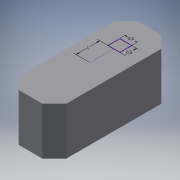
# Autodesk Inventor part: Stiftlist
Saved by Autodesk Inventor 2019 (Build 230136000, 136)
## iProperties
Created: 2018-12-16
Part Number: Stiftlist
Material: Generic
Document SubType Name: Modeling
Designer: Filip
Density: 1 g/cm^3
Appearance: Default
Author: Filip
Autodesk Inventor part; units mm, degrees
ref_plane "YZ Plane" through (0, 0, 0) normal (1, 0, 0) x (0, 1, 0)
ref_plane "XZ Plane" through (0, 0, 0) normal (0, 1, 0) x (-1, 0, 0)
ref_plane "XY Plane" through (0, 0, 0) normal (0, 0, 1) x (1, 0, 0)
sketch "Sketch1" plane through (0, 0, 0) normal (0, 1, 0) x (-1, 0, 0)
  line L0 (-1, -2.5) -> (1, -2.5)
  line L1 (1, -2.5) -> (1, 2.5)
  line L2 (1, 2.5) -> (-1, 2.5)
  line L3 (-1, 2.5) -> (-1, -2.5)
  line L4 (-1, -2.5) -> (1, 2.5) construction
  line L5 (1, -2.5) -> (-1, 2.5) construction
  point P0 (0, 0)
  dimension "d0" = 5
  dimension "d1" = 2
  constraints: 12 end point, 2 midpoint, 2 parallel, 1 horizontal, 1 perpendicular
  measures "d0" distance of L0.end L1.end
  measures "d1" distance of L1.end L2.end
extrude "Extrusion1" add sketch "Sketch1" along normal blind 2
chamfer "Chamfer1" distance 0.5 angle 45 4 edges at (1, 1, 2.5) (-1, 1, 2.5) (1, 1, -2.5) (-1, 1, -2.5)
sketch "Sketch2" plane through (0, 2, 0) normal (0, 1, 0) x (1, 0, 0)
  line L0 (0, 0) -> (0, 1) construction
  line L1 (-0.25, 1) -> (0.25, 1)
  line L2 (0.25, 1) -> (0.25, 1.5)
  line L3 (0.25, 1.5) -> (-0.25, 1.5)
  line L4 (-0.25, 1.5) -> (-0.25, 1)
  line L5 (0, 0) -> (-0.4519, 0) construction
  dimension "d7" = 1
  dimension "d8" = 0.5
  dimension "d9" = 0.5
  constraints: 12 end point, 2 horizontal, 2 parallel, 1 midpoint, 1 perpendicular, 1 vertical
  measures "d7" distance of L0.end L0.start
  measures "d8" distance of L3.end L2.end
  measures "d9" distance of L1.end L2.end
body "Solid1"
